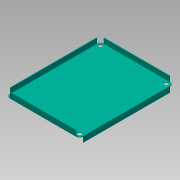
# Autodesk Inventor part: Cart_MID_SHELF
Saved by Autodesk Inventor 2015 (Build 190159000, 159)
## iProperties
Created: 2015-05-21
Part Number: Cart_MID_SHELF
Material: Generic
Document SubType Name: Modeling
Designer: Joe Sheldon
Density: 1 g/cm^3
Appearance: Default
Author: Joe Sheldon
Autodesk Inventor part; units mm, degrees
ref_plane "YZ Plane" through (0, 0, 0) normal (1, 0, 0) x (0, 1, 0)
ref_plane "XZ Plane" through (0, 0, 0) normal (0, 1, 0) x (-1, 0, 0)
ref_plane "XY Plane" through (0, 0, 0) normal (0, 0, 1) x (1, 0, 0)
sketch "Sketch1" plane through (0, 0, 0) normal (0, 1, 0) x (-1, 0, 0)
  line L0 (0, 0) -> (-361.95, 0)
  line L1 (-361.95, 0) -> (-361.95, -463.55)
  line L2 (-361.95, -463.55) -> (0, -463.55)
  line L3 (0, -463.55) -> (0, 0)
  dimension "d0" = 361.95
  dimension "d1" = 463.55
  constraints: 8 end point, 2 parallel, 1 horizontal, 1 perpendicular
  measures "d0" distance of L2.end L1.end
  measures "d1" distance of L1.end L0.end
extrude "Extrusion1" add sketch "Sketch1" along normal blind 2.794
fillet "Fillet1" radius 19.05 4 edges at (361.95, 1.397, 0) (361.95, 1.397, -463.55) (0, 1.397, -463.55) (0, 1.397, 0)
sketch "Sketch3" plane through (0, 0, 0) normal (0, -1, 0) x (1, 0, 0)
  line L0 (361.95, -19.05) -> (359.3341, -19.05)
  line L1 (359.3341, -19.05) -> (359.3341, -444.5)
  line L2 (359.3341, -444.5) -> (361.95, -444.5)
  line L3 (361.95, -444.5) -> (361.95, -19.05)
  point P0 (0, 0)
  constraints: 8 end point, 2 parallel, 1 horizontal, 1 perpendicular
extrude "Extrusion2" add sketch "Sketch3" along normal blind 25.4
sketch "Sketch4" plane through (0, 2.794, 0) normal (0, 1, 0) x (1, 0, 0)
  line L0 (19.05, 0) -> (342.8936, 0)
  line L1 (342.8936, 0) -> (342.8936, 2.7101)
  line L2 (342.8936, 2.7101) -> (19.05, 2.7101)
  line L3 (19.05, 2.7101) -> (19.05, 0)
  line L4 (0, 19.05) -> (2.9466, 19.05)
  line L5 (2.9466, 19.05) -> (2.9466, 444.7516)
  line L6 (2.9466, 444.7516) -> (0, 444.7516)
  line L7 (0, 444.7516) -> (0, 19.05)
  line L8 (342.9, 463.55) -> (19.05, 463.55)
  line L9 (19.05, 463.55) -> (19.05, 460.6098)
  line L10 (19.05, 460.6098) -> (342.9, 460.6098)
  line L11 (342.9, 460.6098) -> (342.9, 463.55)
  point P0 (0, 0)
  constraints: 24 end point, 6 parallel, 3 horizontal, 3 perpendicular
extrude "Extrusion3" add sketch "Sketch4" along normal blind 25.4
sketch "Sketch5" plane through (0, 2.794, 0) normal (0, 1, 0) x (1, 0, 0)
  line L0 (19.05, 460.6098) -> (19.05, 463.55) projected
  arc A0 (19.05, 463.55) -> (0.0017, 444.7516) centre (19.05, 444.5) ccw projected
  line L1 (0.0017, 444.7516) -> (2.9466, 444.7516) projected
  line L2 (2.9466, 444.7516) -> (2.9466, 19.05) projected
  line L3 (2.9466, 19.05) -> (0, 19.05) projected
  arc A1 (0, 19.05) -> (19.05, 0) centre (19.05, 19.05) ccw projected
  line L4 (19.05, 0) -> (19.05, 2.7101) projected
  line L5 (19.05, 2.7101) -> (342.8936, 2.7101) projected
  line L6 (342.8936, 2.7101) -> (342.8936, 0) projected
  line L7 (342.8936, 0) -> (342.9, 0) projected
  arc A2 (342.9, 0) -> (361.95, 19.05) centre (342.9, 19.05) ccw projected
  line L8 (361.95, 19.05) -> (361.95, 444.5) projected
  arc A3 (361.95, 444.5) -> (342.9, 463.55) centre (342.9, 444.5) ccw projected
  line L9 (342.9, 463.55) -> (342.9, 460.6098) projected
  line L10 (342.9, 460.6098) -> (19.05, 460.6098) projected
  circle A4 centre (19.05, 19.05) radius 9.525
  circle A5 centre (19.05, 444.5) radius 9.525
  point P0 (0, 0)
  dimension "d11" = 19.05
  dimension "d12" = 19.05
  constraints: 2 centre point, 2 coincident
  measures "d11" diameter of A4
  measures "d12" diameter of A5
extrude "Extrusion4" cut sketch "Sketch5" against normal blind 25.4 contours A4 | A5
sketch "Sketch6" plane through (0, 2.794, 0) normal (0, 1, 0) x (1, 0, 0)
  circle A0 centre (19.05, 19.05) radius 9.525 projected
  circle A1 centre (19.05, 444.5) radius 9.525 projected
  line L0 (19.05, 460.6098) -> (19.05, 463.55) projected
  arc A2 (19.05, 463.55) -> (0.0017, 444.7516) centre (19.05, 444.5) ccw projected
  line L1 (0.0017, 444.7516) -> (2.9466, 444.7516) projected
  line L2 (2.9466, 444.7516) -> (2.9466, 19.05) projected
  line L3 (2.9466, 19.05) -> (0, 19.05) projected
  arc A3 (0, 19.05) -> (19.05, 0) centre (19.05, 19.05) ccw projected
  line L4 (19.05, 0) -> (19.05, 2.7101) projected
  line L5 (19.05, 2.7101) -> (342.8936, 2.7101) projected
  line L6 (342.8936, 2.7101) -> (342.8936, 0) projected
  line L7 (342.8936, 0) -> (342.9, 0) projected
  arc A4 (342.9, 0) -> (361.95, 19.05) centre (342.9, 19.05) ccw projected
  line L8 (361.95, 19.05) -> (361.95, 444.5) projected
  arc A5 (361.95, 444.5) -> (342.9, 463.55) centre (342.9, 444.5) ccw projected
  line L9 (342.9, 463.55) -> (342.9, 460.6098) projected
  line L10 (342.9, 460.6098) -> (19.05, 460.6098) projected
  circle A6 centre (342.9, 19.05) radius 9.525
  circle A7 centre (342.9, 444.5) radius 9.525
  point P0 (0, 0)
  dimension "d15" = 19.05
  dimension "d16" = 19.05
  constraints: 2 centre point, 2 coincident
  measures "d15" diameter of A6
  measures "d16" diameter of A7
extrude "Extrusion5" cut sketch "Sketch6" against normal blind 25.4 contours A6 | A7
body "Solid1"
